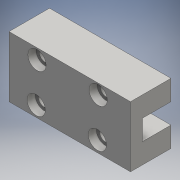
# Autodesk Inventor part: braket1
Saved by Autodesk Inventor 2016 (Build 200138000, 138)
## iProperties
Created: 2016-05-11
Part Number: braket1
Material: 一般
Document SubType Name: Modeling
Designer: 宏太
Density: 1 g/cm^3
Appearance: 既定
Author: 宏太
Autodesk Inventor part; units mm, degrees
ref_plane "YZ Plane" through (0, 0, 0) normal (1, 0, 0) x (0, 1, 0)
ref_plane "XZ Plane" through (0, 0, 0) normal (0, 1, 0) x (-1, 0, 0)
ref_plane "XY Plane" through (0, 0, 0) normal (0, 0, 1) x (1, 0, 0)
sketch "スケッチ1" plane through (0, 0, 0) normal (0, 1, 0) x (-1, 0, 0)
  line L0 (0, 0) -> (30, 0)
  line L1 (30, 0) -> (30, 15)
  line L2 (30, 15) -> (0, 15)
  line L3 (0, 15) -> (0, 0)
  dimension "d0" = 30
  dimension "d1" = 15
  constraints: 8 end point, 2 parallel, 1 horizontal, 1 perpendicular
  measures "d0" distance of L2.end L1.end
  measures "d1" distance of L1.end L0.end
extrude "押し出し1" add sketch "スケッチ1" along normal blind 10
sketch "スケッチ2" plane through (0, 0, 0) normal (1, 0, 0) x (0, 1, 0)
  line L0 (3, 5) -> (10, 5)
  line L1 (10, 5) -> (10, 10)
  line L2 (10, 10) -> (3, 10)
  line L3 (3, 10) -> (3, 5)
  point P0 (0, 0)
  dimension "d4" = 7
  dimension "d5" = 5
  dimension "d6" = 10
  dimension "d7" = 10
  constraints: 8 end point, 2 parallel, 1 horizontal, 1 perpendicular
  measures "d4" distance of L2.end L1.end
  measures "d5" distance of L1.end L0.end
  measures "d6" distance from line of point (0, 0) L1
  measures "d7" distance from line of point (0, 0) L2
extrude "押し出し2" cut sketch "スケッチ2" against normal blind 30
hole "穴1" at (-23.0862, 0, 12.3913) direction (0, 1, 0) diameter 3 depth 10 tip angle 118 counterbore diameter 4.5 counterbore depth 2
hole "穴2" at (-7.9763, 0, 12.4901) direction (0, 1, 0) diameter 3 depth 10 tip angle 118 counterbore diameter 4.5 counterbore depth 2
hole "穴3" at (-23.2858, 0, 2.6671) direction (0, 1, 0) diameter 3 depth 10 tip angle 118 counterbore diameter 4.5 counterbore depth 2
hole "穴4" at (-8.1857, 0, 2.7752) direction (0, 1, 0) diameter 3 depth 10 tip angle 118 counterbore diameter 4.5 counterbore depth 2
